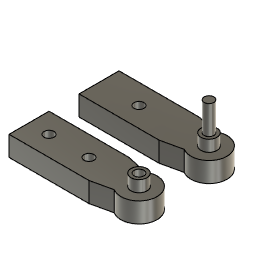
RezacRemeniceZaKais(Untitled) v2 (Autodesk Fusion 360 design; units mm, degrees)
Autodesk Fusion 360 part; units mm, degrees
sketch "Sketch1" plane through (0, 0, 0) normal (0, 0, 1) x (1, 0, 0)
  line L0 (50, 150) -> (50, 130)
  line L1 (50, 150) -> (90, 150)
  line L2 (50, 130) -> (90, 130)
  line L3 (90, 130) -> (100.3351, 132.3033)
  line L4 (90, 150) -> (100.3351, 147.6967)
  arc A0 (100.3351, 132.3033) -> (100.3351, 147.6967) centre (105, 140) ccw
  dimension "d1" = 20
  dimension "d2" = 40
  dimension "d3" = 40
  dimension "d4" = 18
  constraint vertical L0
  constraint perpendicular L0 L1
  constraint perpendicular L0 L2
  measures "d1" distance of L0.start L0.end
  measures "d2" distance of L0.start L1.end
  measures "d3" distance of L0.end L2.end
  measures "d4" diameter of A0
extrude "Extrude1" add sketch "Sketch1" along normal blind 10 makes body 1
sketch "Sketch2" plane through (0, 0, 10) normal (0, 0, 1) x (-1, 0, 0)
  line L0 (-50, -150) -> (-50, -130)
  line L1 (-50, -130) -> (-90, -130)
  line L2 (-90, -130) -> (-100.3351, -132.3033)
  arc A0 (-100.3351, -132.3033) -> (-100.3351, -147.6967) centre (-105, -140) ccw
  line L3 (-100.3351, -147.6967) -> (-90, -150)
  line L4 (-90, -150) -> (-50, -150)
  circle A1 centre (-105, -140) radius 2.45
  circle A2 centre (-105, -140) radius 4
  dimension "d7" = 4.9
  dimension "d8" = 8
  constraint concentric A0 A1
  constraint concentric A1 A2
  measures "d7" diameter of A1
  measures "d8" diameter of A2
extrude "Extrude2" add sketch "Sketch2" along normal blind 20 contours A1 bodies 1
sketch "Sketch3" plane through (0, 0, 10) normal (0, 0, 1) x (-1, 0, 0)
  circle A0 centre (-105, -140) radius 2.45
  line L0 (-50, -150) -> (-50, -130)
  line L1 (-50, -130) -> (-90, -130)
  line L2 (-90, -130) -> (-100.3351, -132.3033)
  arc A1 (-100.3351, -132.3033) -> (-100.3351, -147.6967) centre (-105, -140) ccw
  line L3 (-100.3351, -147.6967) -> (-90, -150)
  line L4 (-90, -150) -> (-50, -150)
  circle A2 centre (-105, -140) radius 4
  dimension "d11" = 8
  constraint concentric A0 A2
  measures "d11" diameter of A2
extrude "Extrude3" add sketch "Sketch3" along normal blind 5.7 contours A2 bodies 1
sketch "Sketch4" plane through (0, 0, 30) normal (0, 0, 1) x (-1, 0, 0)
  circle A0 centre (-105, -140) radius 2.45
  line L0 (-50, -115) -> (-50, -95)
  line L1 (-50, -115) -> (-90, -115)
  line L2 (-50, -95) -> (-90, -95)
  circle A1 centre (-105, -105) radius 4
  circle A2 centre (-105, -105) radius 2.45
  line L3 (-100.3128, -97.3169) -> (-90, -95)
  line L4 (-90, -115) -> (-100.3128, -112.6831)
  arc A3 (-100.3128, -97.3169) -> (-100.3128, -112.6831) centre (-105, -105) ccw
  dimension "d14" = 20
  dimension "d15" = 40
  dimension "d16" = 8
  dimension "d17" = 4.9
  dimension "d18" = 18
  constraint vertical L0
  constraint perpendicular L0 L1
  constraint perpendicular L0 L2
  constraint concentric A1 A2
  constraint concentric A1 A3
  measures "d14" distance of L0.start L0.end
  measures "d15" distance of L0.start L1.end
  measures "d16" diameter of A1
  measures "d17" diameter of A2
  measures "d18" diameter of A3
extrude "Extrude4" add sketch "Sketch4" along normal blind 10 separate body contours L0 L1 L2 L3 L4 A3 | A1 | A2 makes body 2
sketch "Sketch5" plane through (0, 0, 40) normal (0, 0, 1) x (-1, 0, 0)
  line L0 (-50, -115) -> (-50, -95)
  line L1 (-50, -95) -> (-90, -95)
  line L2 (-90, -95) -> (-100.3128, -97.3169)
  arc A0 (-100.3128, -97.3169) -> (-100.3128, -112.6831) centre (-105, -105) ccw
  line L3 (-100.3128, -112.6831) -> (-90, -115)
  line L4 (-90, -115) -> (-50, -115)
  circle A1 centre (-105, -105) radius 2.45
  circle A2 centre (-105, -105) radius 4
  dimension "d21" = 4.9
  dimension "d22" = 8
  constraint concentric A0 A1
  constraint concentric A1 A2
  measures "d21" diameter of A1
  measures "d22" diameter of A2
extrude "Extrude5" add sketch "Sketch5" along normal blind 5.7 contours A2 bodies 2
sketch "Sketch6" plane through (0, 0, 10) normal (0, 0, 1) x (-1, 0, 0)
  circle A0 centre (-105, -140) radius 4
  line L0 (-50, -150) -> (-50, -130)
  line L1 (-50, -130) -> (-90, -130)
  line L2 (-90, -130) -> (-100.3351, -132.3033)
  arc A1 (-100.3351, -132.3033) -> (-100.3351, -147.6967) centre (-105, -140) ccw
  line L3 (-100.3351, -147.6967) -> (-90, -150)
  line L4 (-90, -150) -> (-50, -150)
  circle A2 centre (-70, -140) radius 2.5
  circle A3 centre (-70, -105) radius 2.5
  dimension "d25" = 5
  dimension "d26" = 5
  measures "d25" diameter of A2
  measures "d26" diameter of A3
extrude "Extrude6" cut sketch "Sketch6" against normal blind 35 contours A2 bodies 1
sketch "Sketch7" plane through (0, 0, 40) normal (0, 0, 1) x (-1, 0, 0)
  line L0 (-50, -115) -> (-50, -95)
  line L1 (-50, -95) -> (-90, -95)
  line L2 (-90, -95) -> (-100.3128, -97.3169)
  arc A0 (-100.3128, -97.3169) -> (-100.3128, -112.6831) centre (-105, -105) ccw
  line L3 (-100.3128, -112.6831) -> (-90, -115)
  line L4 (-90, -115) -> (-50, -115)
  circle A1 centre (-105, -105) radius 4
  circle A2 centre (-60, -105) radius 2.5
  circle A3 centre (-80, -105) radius 2.5
  dimension "d29" = 5
  dimension "d30" = 5
  measures "d29" diameter of A2
  measures "d30" diameter of A3
extrude "Extrude7" cut sketch "Sketch7" against normal blind 20 contours A2 | A3 bodies 2
move_body "Move1" bodies 2 to x (1, 0, 0) y (0, 1, 0) z (0, 0, 1) at (0, 0, -30)
